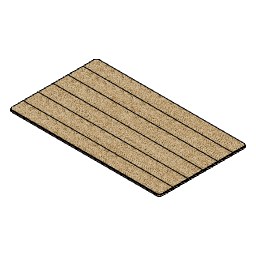
model (Autodesk Fusion 360 design; units mm, degrees)
Autodesk Fusion 360 part; units mm, degrees
sketch "board" plane through (0, 0, 0) normal (0, 0, 1) x (1, 0, 0) in component "top"
  line L0 (0, 0) -> (1222, 0)
  line L1 (1222, 0) -> (1222, 119)
  line L2 (1222, 119) -> (0, 119)
  line L3 (0, 119) -> (0, 0)
  dimension "d8" = 119
  dimension "d9" = 1222
  constraint horizontal L0
  constraint vertical L1
  constraint horizontal L2
  constraint vertical L3
  constraint coincident L0.start L3.end
  measures "d8" distance of L0.start L2.end
  measures "d9" distance of L0.start L0.end
extrude "Extrude1" add sketch "board" along normal blind 19 makes body 1 in component "top"
pattern_linear "R-Pattern1" count 6 spacing 119 along (0, 1, 0) of bodies 1 makes body 2 at (407.3333, 198.3333, 0) makes body 3 at (407.3333, 317.3333, 0) makes body 4 at (407.3333, 436.3333, 0) makes body 5 at (407.3333, 555.3333, 0) makes body 6 at (407.3333, 674.3333, 0) in component "top"
sketch "target" plane through (0, 0, 0) normal (0, 0, 1) x (1, 0, 0) in component "top"
  line L0 (11, 7) -> (1211, 7)
  line L1 (1211, 7) -> (1211, 707)
  line L2 (1211, 707) -> (11, 707)
  line L3 (11, 707) -> (11, 7)
  line L4 (1211, 707) -> (1222, 714) construction
  line L5 (1211, 7) -> (1222, 0) construction
  line L6 (11, 7) -> (0, 0) construction
  line L7 (0, 714) -> (11, 707) construction
  point P0 (1222, 0)
  point P1 (0, 714)
  point P2 (1222, 714)
  dimension "d16" = 1200
  dimension "d17" = 700
  constraint horizontal L0
  constraint vertical L1
  constraint horizontal L2
  constraint vertical L3
  constraint coincident P0 L5.end
  constraint coincident L6.end origin
  constraint coincident P1 L7.start
  constraint equal L4 L5
  constraint equal L4 L7
  constraint equal L6 L7
  constraint coincident P2 L4.end
  measures "d16" distance of L0.start L0.end
  measures "d17" distance of L0.start L2.end
extrude "Extrude2" cut sketch "target" along normal up to surface (19 mm away) keep common part bodies 1 2 3 4 5 6 in component "top"
sketch "top profile" plane through (0, 0, 19) normal (0, 0, 1) x (-1, 0, 0) in component "top"
  line L0 (-11, -119) -> (-11, -7)
  line L1 (-11, -7) -> (-1211, -7)
  line L2 (-1211, -7) -> (-1211, -119)
  line L3 (-1211, -119) -> (-11, -119)
  line L4 (-36, -7) -> (-1186, -7)
  line L5 (-1211, -32) -> (-1211, -682)
  line L6 (-1186, -707) -> (-36, -707)
  line L7 (-11, -682) -> (-11, -32)
  arc A0 (-36, -707) -> (-11, -682) centre (-36, -682) ccw
  arc A1 (-1211, -682) -> (-1186, -707) centre (-1186, -682) ccw
  arc A2 (-1186, -7) -> (-1211, -32) centre (-1186, -32) ccw
  arc A3 (-11, -32) -> (-36, -7) centre (-36, -32) ccw
  line L8 (-1211, -707) -> (-11, -707)
  line L9 (-1211, -7) -> (-1211, -707)
  line L10 (-11, -7) -> (-1211, -7)
  line L11 (-11, -707) -> (-11, -7)
  point P0 (-1211, -707)
  dimension "d21" = 25
  constraint horizontal L4
  constraint vertical L5
  constraint horizontal L6
  constraint vertical L7
  constraint tangent L6 A0
  constraint tangent L7 A0
  constraint tangent L5 A1
  constraint tangent L6 A1
  constraint equal A0 A1
  constraint tangent L4 A2
  constraint tangent L5 A2
  constraint equal A0 A2
  constraint tangent L4 A3
  constraint tangent L7 A3
  constraint equal A0 A3
  constraint collinear L6 L8
  constraint collinear L5 L9
  constraint collinear L4 L10
  constraint collinear L7 L11
  measures "d21" radius of A0
extrude "Extrude3" cut sketch "top profile" against normal up to surface (19 mm away) contours L0 L1 L2 L3 L4 L5 L7 A2 A3 L9 L10 L11 | L3 L5 L6 L7 A0 A1 L8 L9 L11 keep common part bodies 1 2 3 4 5 6 in component "top"
fillet "Fillet1" radius 3.175 18 edges at (1211, 75.5, 19) (1203.6777, 14.3223, 19) (611, 7, 19) (18.3223, 14.3223, 19) (11, 75.5, 19) (1211, 178.5, 19) (11, 178.5, 19) (1211, 297.5, 19) (11, 297.5, 19) (1211, 416.5, 19) (11, 416.5, 19) (1211, 535.5, 19) (11, 535.5, 19) (11, 638.5, 19) (18.3223, 699.6777, 19) (611, 707, 19) (1203.6777, 699.6777, 19) (1211, 638.5, 19) on bodies 1 2 3 4 5 6 in component "top"
chamfer "Chamfer1" distance 6.3333 angle 45 18 edges at (1211, 416.5, 0) (11, 416.5, 0) (1211, 297.5, 0) (11, 297.5, 0) (611, 7, 0) (18.3223, 14.3223, 0) (11, 75.5, 0) (1211, 75.5, 0) (1203.6777, 14.3223, 0) (1211, 178.5, 0) (11, 178.5, 0) (1211, 638.5, 0) (1203.6777, 699.6777, 0) (611, 707, 0) (18.3223, 699.6777, 0) (11, 638.5, 0) (1211, 535.5, 0) (11, 535.5, 0) on bodies 1 2 3 4 5 6 in component "top"
sketch "hardware" plane through (0, 0, 0) normal (0, 0, 1) x (1, 0, 0) in component "hardware"
  line L0 (36, 17) -> (61, 17)
  line L1 (61, 17) -> (61, 697)
  line L2 (61, 697) -> (36, 697)
  line L3 (36, 697) -> (36, 17)
  line L4 (11, 707) -> (11, 7)
  line L5 (11, 7) -> (1211, 7)
  line L6 (1211, 707) -> (11, 707)
  line L7 (1211, 7) -> (1211, 707) construction
  line L8 (11, 357) -> (1211, 357) construction
  line L9 (611, 7) -> (611, 707) construction
  line L10 (1186, 697) -> (1186, 17)
  line L11 (1186, 17) -> (1161, 17)
  line L12 (1161, 697) -> (1186, 697)
  line L13 (1161, 17) -> (1161, 697)
  line L14 (137.2, 52.2) -> (213.4, 52.2)
  line L15 (213.4, 52.2) -> (213.4, 661.8)
  line L16 (213.4, 661.8) -> (137.2, 661.8)
  line L17 (137.2, 661.8) -> (137.2, 52.2)
  line L18 (175.3, 52.2) -> (175.3, 661.8) construction
  line L19 (137.2, 52.2) -> (213.4, 174.12) construction
  line L20 (213.4, 174.12) -> (137.2, 174.12) construction
  line L21 (137.2, 174.12) -> (213.4, 296.04) construction
  line L22 (213.4, 296.04) -> (137.2, 296.04) construction
  line L23 (137.2, 296.04) -> (213.4, 417.96) construction
  line L24 (213.4, 417.96) -> (137.2, 417.96) construction
  line L25 (137.2, 417.96) -> (213.4, 539.88) construction
  line L26 (213.4, 539.88) -> (137.2, 539.88) construction
  line L27 (137.2, 539.88) -> (213.4, 661.8) construction
  circle A0 centre (175.3, 174.12) radius 3.5
  circle A1 centre (175.3, 296.04) radius 3.5
  circle A2 centre (175.3, 417.96) radius 3.5
  circle A3 centre (175.3, 539.88) radius 3.5
  line L28 (1084.8, 661.8) -> (1084.8, 52.2)
  line L29 (1084.8, 52.2) -> (1008.6, 52.2)
  line L30 (1008.6, 661.8) -> (1084.8, 661.8)
  line L31 (1008.6, 52.2) -> (1008.6, 661.8)
  circle A4 centre (1046.7, 539.88) radius 3.5
  circle A5 centre (1046.7, 417.96) radius 3.5
  circle A6 centre (1046.7, 174.12) radius 3.5
  circle A7 centre (1046.7, 296.04) radius 3.5
  point P0 (175.3, 357)
  dimension "d24" = 25
  dimension "d25" = 10
  dimension "d26" = 10
  dimension "d27" = 25
  dimension "d28" = 609.6
  dimension "d29" = 76.2
  dimension "d30" = 7
  dimension "d31" = 76.2
  constraint horizontal L0
  constraint vertical L1
  constraint horizontal L2
  constraint vertical L3
  constraint midpoint L4 L8.start
  constraint midpoint L7 L8.end
  constraint midpoint L5 L9.start
  constraint midpoint L6 L9.end
  constraint symmetric L0.start L9 L10.end
  constraint symmetric L0.end L9 L11.end
  constraint symmetric L1.end L9 L12.start
  constraint symmetric L2.end L9 L10.start
  constraint horizontal L14
  constraint vertical L15
  constraint horizontal L16
  constraint vertical L17
  constraint midpoint L14 L18.start
  constraint midpoint L16 L18.end
  constraint midpoint L18 P0
  constraint coincident L8 P0
  constraint coincident L15 L19.end
  constraint coincident L17 L20.end
  constraint perpendicular L17 L20
  constraint coincident L15 L21.end
  constraint coincident L17 L22.end
  constraint perpendicular L17 L22
  constraint coincident L15 L23.end
  constraint coincident L17 L24.end
  constraint perpendicular L17 L24
  constraint coincident L15 L25.end
  constraint coincident L17 L26.end
  constraint perpendicular L17 L26
  constraint equal L19 L21
  constraint equal L21 L23
  constraint equal L23 L25
  constraint equal L25 L27
  constraint midpoint L20 A0.centre
  constraint midpoint L22 A1.centre
  constraint midpoint L24 A2.centre
  constraint midpoint L26 A3.centre
  constraint equal A0 A1
  constraint equal A1 A2
  constraint equal A2 A3
  constraint symmetric L9 L14.start L28.end
  constraint symmetric L9 L14.end L29.end
  constraint symmetric L9 L15.end L30.start
  constraint symmetric L9 L16.end L28.start
  constraint symmetric L9 A0 A6
  constraint symmetric L9 A1 A7
  constraint symmetric L9 A2 A5
  constraint symmetric L9 A3 A4
  measures "d24" distance of L3 L4
  measures "d25" distance of L0 L5
  measures "d26" distance of L2 L6
  measures "d27" distance of L1 L3
  measures "d28" distance of L14.start L16.end
  measures "d29" distance of L14.start L14.end
  measures "d30" diameter of A0
  measures "d31" distance of L1 L17
component "top" placed x (1, 0, 0) y (0, 1, 0) z (0, 0, 1) at (0, 0, 0)
component "hardware" placed x (1, 0, 0) y (0, 1, 0) z (0, 0, 1) at (0, 0, 0)
equation "rawBoardWidth = 129 mm"
equation "boardThickness = 19 mm"
equation "boardLength = 1222 mm"
equation "boardWidth = rawBoardWidth - ( 2 * 5 ) * 1 mm"
equation "targetWidth = 1200 mm"
equation "targetDepth = 700 mm"
equation "boardCount = 6"
equation "d8 = boardWidth"
equation "d9 = boardLength"
equation "d10 = boardThickness"
equation "d12 = boardCount"
equation "d14 = boardWidth"
equation "d16 = targetWidth"
equation "d17 = targetDepth"
equation "cornerRadius = 25 mm"
equation "d21 = cornerRadius"
equation "d26 = d25"
equation "d28 = 24\""
equation "d29 = 3\""
equation "d31 = d29"
equation "d33 = 1/8\""
equation "d34 = boardThickness / 3"
